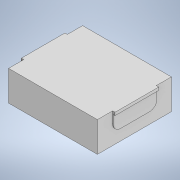
# Autodesk Inventor part: iRobot_filter
Saved by Autodesk Inventor 2020 (Build 240168000, 168)
## iProperties
Created: 2020-04-05
Part Number: iRobot_filter
Material: Generic
Document SubType Name: Modeling
Designer: Clevo
Density: 1 g/cm^3
Appearance: Default
Author: Clevo
Autodesk Inventor part; units mm, degrees
ref_plane "YZ Plane" through (0, 0, 0) normal (1, 0, 0) x (0, 1, 0)
ref_plane "XZ Plane" through (0, 0, 0) normal (0, 1, 0) x (-1, 0, 0)
ref_plane "XY Plane" through (0, 0, 0) normal (0, 0, 1) x (1, 0, 0)
sketch "Sketch1" plane through (0, 0, 0) normal (0, 1, 0) x (-1, 0, 0)
  line L0 (-30.48, -25.4) -> (30.48, -25.4)
  line L1 (30.48, -25.4) -> (30.48, 25.4)
  line L2 (30.48, 25.4) -> (-30.48, 25.4)
  line L3 (-30.48, 25.4) -> (-30.48, -25.4)
  line L4 (-30.48, -25.4) -> (30.48, 25.4) construction
  line L5 (30.48, -25.4) -> (-30.48, 25.4) construction
  point P0 (0, 0)
  dimension "d0" = 50.8
  dimension "d1" = 60.96
  constraints: 12 end point, 2 midpoint, 2 parallel, 1 horizontal, 1 perpendicular
  measures "d0" distance of L0.end L1.end
  measures "d1" distance of L1.end L2.end
extrude "Extrusion1" add sketch "Sketch1" along normal blind 20.6629
sketch "Sketch2" plane through (30.48, 0, 25.4) normal (1, 0, 0) x (0, 0, -1)
  line L0 (0, 0) -> (50.8, 0) projected
  line L1 (50.8, 0) -> (50.8, 20.6629) projected
  line L2 (0, 20.6629) -> (50.8, 20.6629) projected
  line L3 (0, 0) -> (0, 20.6629) projected
  line L4 (0, 20.6629) -> (50.8, 20.6629) projected
  line L5 (10.4, 20.6629) -> (40.4, 20.6629)
  line L6 (40.4, 20.6629) -> (40.4, 7.9629)
  line L7 (40.4, 7.9629) -> (10.4, 7.9629)
  line L8 (10.4, 7.9629) -> (10.4, 20.6629)
  point P0 (25.4, 0)
  point P1 (25.4, 20.6629)
  point P2 (25.4, 20.6629)
  point P3 (10.4, 20.6629)
  dimension "d4" = 12.7
  dimension "d5" = 30
  constraints: 8 end point, 2 midpoint, 2 parallel, 1 coincident, 1 horizontal, 1 perpendicular, 1 point on line
  measures "d4" distance of L5.end L6.end
  measures "d5" distance of L6.end L7.end
extrude "Extrusion2" add sketch "Sketch2" along normal blind 0.5 contours L2 L6 L7 L8
fillet "Fillet1" radius 5 2 edges at (30.73, 7.9629, 15) (30.73, 7.9629, -15)
sketch "Sketch3" plane through (30.98, 0, 25.4) normal (1, 0, 0) x (0, 0, -1)
  arc A0 (35.4, 7.9629) -> (40.4, 12.9629) centre (35.4, 12.9629) ccw projected
  line L0 (40.4, 12.9629) -> (40.4, 20.6629) projected
  line L1 (40.4, 20.6629) -> (10.4, 20.6629) projected
  line L2 (10.4, 20.6629) -> (10.4, 12.9629) projected
  arc A1 (10.4, 12.9629) -> (15.4, 7.9629) centre (15.4, 12.9629) ccw projected
  line L3 (15.4, 7.9629) -> (35.4, 7.9629) projected
  line L4 (40.4, 20.6629) -> (10.4, 20.6629) projected
  line L5 (40.4, 12.9629) -> (40.4, 20.6629) projected
  line L6 (10.4, 20.6629) -> (40.4, 20.6629)
  line L7 (40.4, 20.6629) -> (40.4, 18.6629)
  line L8 (40.4, 18.6629) -> (10.4, 18.6629)
  line L9 (10.4, 18.6629) -> (10.4, 20.6629)
  point P0 (25.4, 0)
  point P1 (10.4, 18.6629)
  dimension "d9" = 2
  constraints: 8 end point, 2 parallel, 1 horizontal, 1 perpendicular, 1 point on line
  measures "d9" distance between parallel lines of L1 L8
extrude "Extrusion3" add sketch "Sketch3" along normal blind 1.17 contours L8 L2 L1 L0
mirror "Mirror1" about plane through (0, 0, 0) normal (1, 0, 0) of "Extrusion2", "Fillet1", "Extrusion3"
body "Solid1"
